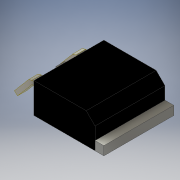
# Autodesk Inventor part: TN2540-800G-TR
Saved by Autodesk Inventor 2017 (Build 210142000, 142)
## iProperties
Part Number: TN2540-800G-TR
Material: Generisch
Document SubType Name: Modeling
Designer: Philomena-Theresa
Density: 1 g/cm^3
Appearance: Vorgabe
Author: Philomena-Theresa
Autodesk Inventor part; units mm, degrees
ref_plane "YZ Plane" through (0, 0, 0) normal (1, 0, 0) x (0, 1, 0)
ref_plane "XZ Plane" through (0, 0, 0) normal (0, 1, 0) x (-1, 0, 0)
ref_plane "XY Plane" through (0, 0, 0) normal (0, 0, 1) x (1, 0, 0)
sketch "Skizze1" plane through (0, 0, 0) normal (0, 0, 1) x (1, 0, 0)
  line L0 (-5.15, 5.15) -> (5.15, 5.15)
  line L1 (5.15, 5.15) -> (5.15, -5.15)
  line L2 (5.15, -5.15) -> (-5.15, -5.15)
  line L3 (-5.15, -5.15) -> (-5.15, 5.15)
  line L4 (-5.15, 5.15) -> (5.15, -5.15) construction
  point P0 (0, 0)
  point P1 (0, 0)
  dimension "d0" = 10.3
  dimension "d1" = 10.3
  constraints: 10 end point, 2 parallel, 1 coincident, 1 horizontal, 1 midpoint, 1 perpendicular
  measures "d0" distance of L1.end L2.end
  measures "d1" distance of L0.end L1.end
extrude "Extrusion1" add sketch "Skizze1" along normal blind 1.3
sketch "Skizze2" plane through (0, 0, 1.3) normal (0, 0, 1) x (1, 0, 0)
  line L0 (5.15, 5.15) -> (-5.15, 5.15) projected
  line L1 (-5.15, 5.15) -> (3.85, 5.15)
  line L2 (3.85, 5.15) -> (3.85, -5.15)
  line L3 (3.85, -5.15) -> (-5.15, -5.15)
  line L4 (-5.15, -5.15) -> (-5.15, 5.15)
  point P0 (0, 0)
  dimension "d4" = 9
  dimension "d5" = 10.3
  constraints: 8 end point, 2 parallel, 1 horizontal, 1 perpendicular
  measures "d4" distance of L2.end L3.end
  measures "d5" distance of L1.end L2.end
extrude "Extrusion2" add sketch "Skizze2" along normal blind 3.16
chamfer "Fase1" distance 1.3 angle 45 1 edges at (3.85, 0, 4.46)
sketch "Skizze3" plane through (-5.15, -5.15, 0) normal (0, -1, 0) x (1, 0, 0)
  line L0 (10.3, 1.3) -> (9, 1.3) projected
  line L1 (0, 0) -> (10.3, 0) projected
  line L2 (9, 1.3) -> (10.3, 1.3)
  line L3 (10.3, 1.3) -> (10.3, 0)
  line L4 (10.3, 0) -> (9, 0)
  line L5 (9, 0) -> (9, 1.3)
  point P0 (5.15, 0)
  constraints: 8 end point, 2 parallel, 1 horizontal, 1 perpendicular
extrude "Extrusion3" cut sketch "Skizze3" against normal blind 0.001
sketch "Skizze4" plane through (-5.15, 5.15, 0) normal (0, 1, 0) x (1, 0, 0)
  line L0 (9, 0) -> (9, -1.3) projected
  line L1 (10.3, -1.3) -> (10.3, 0) projected
  line L2 (9, -1.3) -> (10.3, -1.3)
  line L3 (10.3, -1.3) -> (10.3, 0)
  line L4 (10.3, 0) -> (9, 0)
  line L5 (9, 0) -> (9, -1.3)
  point P0 (5.15, 0)
  constraints: 8 end point, 2 parallel, 1 horizontal, 1 perpendicular
extrude "Extrusion4" cut sketch "Skizze4" against normal blind 0.001
sketch "Skizze7" plane through (-5.15, -5.15, 0) normal (-1, 0, 0) x (0, 0, 1)
  line L0 (4.46, 10.3) -> (4.46, 0) construction
  line L1 (4.46, 10.3) -> (4.46, 9.1) construction
  line L2 (4.46, 9.1) -> (3.14, 9.1) construction
  line L3 (3.14, 9.1) -> (2.59, 9.1)
  line L4 (2.59, 9.1) -> (2.59, 7.7)
  line L5 (2.59, 7.7) -> (3.14, 7.7)
  line L6 (3.14, 7.7) -> (3.14, 9.1)
  line L7 (0, 0) -> (4.46, 0) construction
  line L8 (4.46, 0) -> (4.46, 1.2) construction
  line L9 (4.46, 1.2) -> (3.14, 1.2) construction
  line L10 (3.14, 1.2) -> (2.59, 1.2)
  line L11 (2.59, 1.2) -> (2.59, 2.6)
  line L12 (2.59, 2.6) -> (3.14, 2.6)
  line L13 (3.14, 2.6) -> (3.14, 1.2)
  point P0 (0, 5.15)
  point P1 (0, 10.3)
  dimension "d20" = 1.2
  dimension "d21" = 1.32
  dimension "d22" = 0.55
  dimension "d23" = 1.4
  dimension "d24" = 1.2
  dimension "d25" = 1.32
  constraints: 24 end point, 4 parallel, 4 perpendicular, 2 equal length, 2 horizontal, 2 point on line
  measures "d20" distance of L0.start L1.end
  measures "d21" distance of L1.end L2.end
  measures "d22" distance of L5.end L4.end
  measures "d23" distance of L4.end L3.end
  measures "d24" distance of L0.end L8.end
  measures "d25" distance of L8.end L9.end
extrude "Extrusion5" add sketch "Skizze7" along normal blind 1.5 separate body
sketch "Skizze9" plane through (-5.15, -3.95, 2.59) normal (0, -1, 0) x (1, 0, 0)
  line L0 (-1.5, 0) -> (-1.5, 0.55) projected
  line L1 (-1.5, 0) -> (-3.6043, -2.4791)
  line L2 (-3.6043, -2.4791) -> (-4.0859, -2.0703)
  line L3 (-4.0859, -2.0703) -> (-1.9816, 0.4088)
  line L4 (-1.9816, 0.4088) -> (-1.5, 0)
  line L5 (-1.5, 0.55) -> (-1.9816, 0.4088)
  line L6 (-1.9816, 0.4088) -> (-1.8331, -0.0977)
  line L7 (-1.8331, -0.0977) -> (-1.3515, 0.0435)
  line L8 (-1.3515, 0.0435) -> (-1.5, 0.55)
  point P0 (5.15, -2.59)
  constraints: 16 end point, 4 parallel, 2 perpendicular
extrude "Extrusion6" add sketch "Skizze9" against normal blind 1.4 contours L4 L5 L0 | L7 L6 L4 | L1 L2 L3 L6 L7 bodies 2
sketch "Skizze11" plane through (-5.15, 2.55, 2.59) normal (0, -1, 0) x (1, 0, 0)
  line L0 (-1.5, 0) -> (-1.5, 0.55)
  line L1 (-1.5, 0) -> (-3.6043, -2.4791)
  line L2 (-3.6043, -2.4791) -> (-4.0859, -2.0703)
  line L3 (-4.0859, -2.0703) -> (-1.9816, 0.4088)
  line L4 (-1.9816, 0.4088) -> (-1.5, 0)
  line L5 (-1.5, 0.55) -> (-1.9816, 0.4088)
  line L6 (-1.9816, 0.4088) -> (-1.8331, -0.0977)
  line L7 (-1.8331, -0.0977) -> (-1.3515, 0.0435)
  line L8 (-1.3515, 0.0435) -> (-1.5, 0.55)
  point P0 (5.15, -2.59)
  constraints: 18 end point, 4 parallel, 2 perpendicular
extrude "Extrusion8" add sketch "Skizze11" against normal blind 1.4 contours L4 L5 L0 | L7 L6 L4 | L1 L2 L3 L6 L7 bodies 2
sketch "Skizze12" plane through (-5.15, -5.15, 0) normal (-1, 0, 0) x (0, 0, 1)
  line L0 (2.59, 7.7) -> (3.14, 7.7) projected
  line L1 (2.865, 7.7) -> (2.865, 6.02) construction
  line L2 (2.865, 7.7) -> (4.545, 7.7) construction
  line L3 (3.14, 6.02) -> (2.59, 6.02)
  line L4 (2.59, 6.02) -> (2.59, 4.72)
  line L5 (2.59, 4.72) -> (3.14, 4.72)
  line L6 (3.14, 4.72) -> (3.14, 6.02)
  point P0 (0, 5.15)
  dimension "d40" = 1.68
  dimension "d41" = 90
  dimension "d42" = 0.55
  dimension "d43" = 1.3
  constraints: 12 end point, 2 horizontal, 2 midpoint, 2 parallel, 2 perpendicular, 1 vertical
  measures "d40" distance of L1.end L1.start
  measures "d41" angle of L1 L2
  measures "d42" distance of L5.end L4.end
  measures "d43" distance of L4.end L3.end
extrude "Extrusion9" add sketch "Skizze12" along normal blind 1.5 bodies 1
